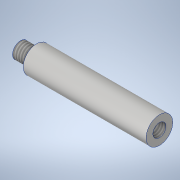
# Autodesk Inventor part: kicker_mitte_alt
Saved by Autodesk Inventor 2020 (Build 240168000, 168)
## iProperties
Part Number: kicker_mitte_alt
Material: Aluminium 6061
Document SubType Name: Modeling
Designer: rYan
Mass: 11.5234 g
Surface Area: 21.4483 cm^2
Volume: 4.26791 cm^3
Density: 2.7 g/cm^3
Appearance: Aluminium - flach
Author: rYan
Autodesk Inventor part; units mm, degrees
ref_plane "YZ Plane" through (0, 0, 0) normal (1, 0, 0) x (0, 1, 0)
ref_plane "XZ Plane" through (0, 0, 0) normal (0, 1, 0) x (-1, 0, 0)
ref_plane "XY Plane" through (0, 0, 0) normal (0, 0, 1) x (1, 0, 0)
sketch "Skizze1" plane through (0, 0, 0) normal (0, 0, 1) x (1, 0, 0)
  line L0 (0, 0) -> (52, 0)
  line L1 (0, 0) -> (0, 3)
  line L2 (0, 3) -> (6, 3)
  line L3 (6, 3) -> (6, 5)
  line L4 (6, 5) -> (52, 5)
  line L5 (52, 5) -> (52, 0)
  dimension "d1" = 6
  dimension "d2" = 10
  dimension "d3" = 6
  dimension "d18" = 52
  constraints: 12 end point, 2 perpendicular, 2 vertical, 1 coincident, 1 horizontal, 1 parallel
  measures "d1" diameter of L2 L0
  measures "d2" diameter of L4 L0
  measures "d3" distance of L1.end L2.end
  measures "d18" distance between parallel lines of L1 L5
revolve "Umdrehung1" add sketch "Skizze1" angle 360 about axis through (0, 0, 0) along (1, 0, 0)
sketch "Skizze2" plane through (52, 0, 0) normal (1, 0, 0) x (0, 0, -1)
  point P0 (0, 0)
  point P1 (0, 0)
  constraints: 1 coincident
hole "Bohrung1" at (52, 0, 0) direction (-1, 0, 0) diameter 4.917 depth 13 tip angle 118 thread size "M6x1" class "6H" standard "ISO Metric profile"
thread "Gewinde1" size "M6x1" class "6g" standard "ANSI Metric M Profile" full length
